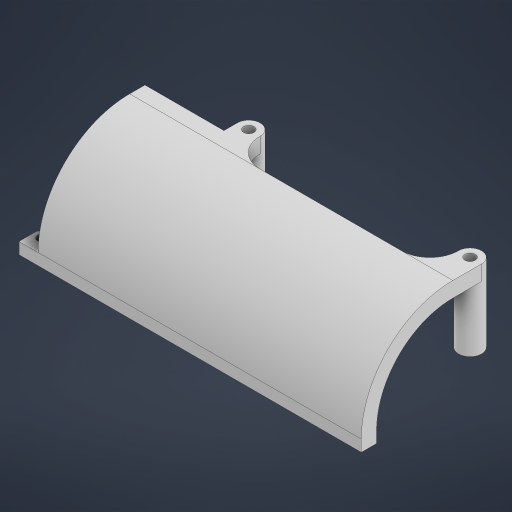
# Autodesk Inventor part: horizental blade
Saved by Autodesk Inventor 2024 (Build 280153000, 153)
## iProperties
Created: 2023-07-13
Part Number: horizental blade
Material: 일반
Document SubType Name: Modeling
Designer: 6gioc
Density: 1 g/cm^3
Appearance: 기본값
Author: 6gioc
Autodesk Inventor part; units mm, degrees
ref_plane "YZ Plane" through (0, 0, 0) normal (1, 0, 0) x (0, 1, 0)
ref_plane "XZ Plane" through (0, 0, 0) normal (0, 1, 0) x (-1, 0, 0)
ref_plane "XY Plane" through (0, 0, 0) normal (0, 0, 1) x (1, 0, 0)
sketch "스케치1" plane through (0, 0, 0) normal (0, 1, 0) x (-1, 0, 0)
  circle A0 centre (0, 0) radius 1.5
  circle A1 centre (0, 0) radius 2.5
  line L0 (2.5, 0) -> (2.5, 4)
  line L1 (2.5, 4) -> (-82.5, 4)
  line L2 (-82.5, 4) -> (-82.5, 0)
  line L3 (-82.5, 0) -> (-2.5, 0)
  line L4 (0, -2.5) -> (-5, -2.5)
  line L5 (-5, -2.5) -> (-7.5, 0)
  dimension "d0" = 3
  dimension "d1" = 5
  dimension "d2" = 4
  dimension "d3" = 85
  dimension "d4" = 5
  dimension "d5" = 135
  constraints: 12 end point, 3 perpendicular, 3 point on circle, 2 centre point, 2 coincident, 2 tangent, 1 horizontal, 1 point on line, 1 vertical
  measures "d0" diameter of A0
  measures "d1" diameter of A1
  measures "d2" distance of L0.start L0.end
  measures "d3" distance of L0.end L1.end
  measures "d4" distance of L4.start L4.end
  measures "d5" angle of L4 L5
extrude "돌출1" add sketch "스케치1" along normal blind 3
sketch "스케치2" plane through (82.5, 0, 4) normal (1, 0, 0) x (0, 0, -1)
  line L0 (4, 3) -> (24, 3)
  arc A0 (24, 27) -> (0, 3) centre (24, 3) ccw
  arc A1 (24, 23) -> (4, 3) centre (24, 3) ccw
  line L1 (24, 27) -> (24, 23)
  line L2 (0, 0) -> (4, 0) projected
  line L3 (4, 0) -> (4, 3) projected
  line L4 (0, 3) -> (4, 3) projected
  line L5 (0, 0) -> (0, 3) projected
  point P0 (4, 0)
  point P1 (0, 3)
  point P2 (4, 3)
  dimension "d8" = 20
  constraints: 4 end point, 4 point on circle, 2 centre point, 2 coincident, 1 horizontal
  measures "d8" distance of L0.start L0.end
extrude "돌출2" add sketch "스케치2" against normal blind 80 contours L1 A1 L4 A0
sketch "스케치3" plane through (82.5, 0, 4) normal (1, 0, 0) x (0, 0, -1)
  line L0 (0, 0) -> (4, 0) projected
  line L1 (4, 0) -> (4, 3) projected
  arc A0 (24, 23) -> (4, 3) centre (24, 3) ccw projected
  line L2 (24, 23) -> (24, 27) projected
  arc A1 (24, 27) -> (0, 3) centre (24, 3) ccw projected
  line L3 (0, 0) -> (0, 3) projected
  point P0 (4, 0)
extrude "돌출3" add sketch "스케치3" along normal blind 4.7
sketch "스케치4" plane through (2.5, 23, -20) normal (0, 0, -1) x (-1, 0, 0)
  line L0 (0, 4) -> (-84.7, 4) projected
  line L1 (-84.7, 4) -> (-78.7, 4)
  line L2 (-78.7, 4) -> (-78.7, 0)
  line L3 (-78.7, 0) -> (-84.7, 0)
  line L4 (-84.7, 0) -> (-84.7, 4)
  point P0 (2.5, -23)
  dimension "d16" = 6
  dimension "d17" = 4
  constraints: 8 end point, 2 parallel, 1 horizontal, 1 perpendicular
  measures "d16" distance of L2.end L3.end
  measures "d17" distance of L1.end L2.end
extrude "돌출4" add sketch "스케치4" along normal blind 10.5
sketch "스케치5" plane through (81.2, 23, -20) normal (0, -1, 0) x (1, 0, 0)
  circle A0 centre (3, -7.5) radius 1.35
  circle A1 centre (3, -7.5) radius 3
  line L0 (0, 0) -> (6, 0) projected
  line L1 (0, 0) -> (0, -10.5) projected
  line L2 (6, -10.5) -> (0, -10.5) projected
  line L3 (6, 0) -> (6, -10.5) projected
  line L4 (6, -10.5) -> (0, -10.5) projected
  line L5 (0, 0) -> (0, -10.5) projected
  point P0 (-81.2, 20)
  dimension "d20" = 2.7
  dimension "d21" = 6
  constraints: 2 centre point, 2 tangent, 1 coincident
  measures "d20" diameter of A0
  measures "d21" diameter of A1
extrude "돌출5" add sketch "스케치5" along normal blind 16.42 contours A1
fillet "모깎기1" radius 3 2 edges at (87.2, 25, -30.5) (81.2, 25, -30.5)
fillet "모깎기2" radius 7.5 1 edges at (81.2, 25, -20)
extrude "돌출6" cut sketch "스케치5" against normal blind 16.42 contours A0
sketch "스케치6" plane through (73.7, 23, -20) normal (0, 0, -1) x (-1, 0, 0)
  line L0 (71.2, 4) -> (0, 4) projected
  line L1 (50.5, 4) -> (44.5, 4)
  line L2 (44.5, 4) -> (44.5, 0)
  line L3 (44.5, 0) -> (50.5, 0)
  line L4 (50.5, 0) -> (50.5, 4)
  line L5 (-11.85, 4) -> (-9.15, 4) projected
  point P0 (73.7, -23)
  point P1 (51.2, 4)
  point P2 (47.5, 4)
  point P3 (-10.5, 4)
  point P4 (44.5, 4)
  dimension "d29" = 6
  dimension "d30" = 4
  dimension "d31" = 58
  constraints: 8 end point, 2 midpoint, 2 parallel, 1 horizontal, 1 perpendicular, 1 point on line
  measures "d29" distance of L3.end L2.end
  measures "d30" distance of L2.end L1.end
  measures "d31" distance of point (47.5, 4) point (-10.5, 4)
extrude "돌출7" add sketch "스케치6" along normal blind 10.5
sketch "스케치7" plane through (23.2, 27, -20) normal (0, 1, 0) x (1, 0, 0)
  circle A0 centre (3, 7.5) radius 1.35
  circle A1 centre (3, 7.5) radius 3
  line L0 (0, 0) -> (0, 10.5) projected
  line L1 (0, 10.5) -> (6, 10.5) projected
  point P0 (-23.2, -20)
  dimension "d34" = 2.7
  dimension "d35" = 6
  constraints: 2 centre point, 2 tangent, 1 coincident
  measures "d34" diameter of A0
  measures "d35" diameter of A1
extrude "돌출8" add sketch "스케치7" against normal blind 20.42 contours A1
extrude "돌출9" cut sketch "스케치7" against normal blind 20.42 contours A0
fillet "모깎기4" radius 3 2 edges at (23.2, 25, -30.5) (29.2, 25, -30.5)
fillet "모깎기6" radius 7.5 1 edges at (29.2, 25, -20)
sketch "스케치8" plane through (2.5, 23, -20) normal (0, 0, -1) x (-1, 0, 0)
  line L0 (-20.7, 4) -> (-20.7, 0) projected
  line L1 (0, 0) -> (-20.7, 0) projected
  line L2 (0, 4) -> (0, 0) projected
  line L3 (0, 4) -> (-20.7, 4) projected
  point P0 (2.5, -23)
extrude "돌출10" add sketch "스케치8" along normal blind 4
sketch "스케치9" plane through (2.5, 23, -20) normal (0, -1, 0) x (1, 0, 0)
  line L0 (0, -4) -> (20.7, -4) projected
  line L1 (0, -4) -> (20.7, -4)
  line L2 (20.7, -4) -> (20.7, -1)
  line L3 (20.7, -1) -> (0, -1)
  line L4 (0, -1) -> (0, -4)
  circle A0 centre (23.7, -7.5) radius 3 projected
  line L5 (25.6463, -5.2171) -> (20.7, -1)
  arc A1 (26.7, -7.5) -> (20.7, -7.5) centre (23.7, -7.5) ccw projected
  arc A2 (34.2, 0) -> (26.7, -7.5) centre (34.2, -7.5) ccw projected
  line L6 (0, 0) -> (34.2, 0) projected
  line L7 (0, 0) -> (0, -4) projected
  line L8 (20.7, -4) -> (0, -4) projected
  line L9 (20.7, -4) -> (20.7, -7.5) projected
  point P0 (-2.5, 20)
  dimension "d45" = 3
  constraints: 10 end point, 2 parallel, 1 horizontal, 1 perpendicular, 3 other
  measures "d45" distance of L2.end L0.end
extrude "돌출11" add sketch "스케치9" along normal blind 16.42 contours L4 L3 L2 L0
sketch "스케치10" plane through (2.5, 0, 4) normal (-1, 0, 0) x (0, 0, 1)
  arc A0 (0, 3) -> (-24, 27) centre (-24, 3) ccw projected
  line L0 (-24, 27) -> (-28, 27) projected
  line L1 (-24, 23) -> (-25, 23) projected
  arc A1 (-4, 3) -> (-24, 23) centre (-24, 3) ccw projected
  line L2 (-28, 27) -> (-28, 6.58) projected
  line L3 (-25, 6.58) -> (-28, 6.58) projected
  line L4 (-25, 23) -> (-25, 6.58) projected
  line L5 (-25, 6.58) -> (-4.2263, 6)
  line L6 (-25, 6.58) -> (-25, 0)
  line L7 (-25, 6.58) -> (-18.42, 6.58) construction
  line L8 (-4, 0) -> (-4, 3) projected
  line L9 (-25, 0) -> (-4, 0)
  arc A2 (-4, 3) -> (-24, 23) centre (-24, 3) ccw projected
  arc A3 (-4, 3) -> (-24, 23) centre (-24, 3) ccw projected
  line L10 (0, 3) -> (-4, 3) projected
  point P0 (-4, 3)
  point P1 (-4.2263, 6)
  dimension "d50" = 90
  constraints: 8 end point, 2 perpendicular, 1 horizontal
  measures "d50" angle of L6 L7
extrude "돌출12" add sketch "스케치10" against normal blind 3 contours L5 L4 L1 A1
sketch "스케치13" plane through (0, 3, 0) normal (0, 1, 0) x (1, 0, 0)
  line L0 (2.5, 0) -> (7.5, 0) projected
  line L1 (7.5, 0) -> (5, 2.5) projected
  line L2 (5, 2.5) -> (0, 2.5) projected
  arc A0 (0, 2.5) -> (-2.5, 0) centre (0, 0) ccw projected
  line L3 (-2.5, 0) -> (-2.5, -4) projected
  line L4 (-2.5, -4) -> (2.5, -4) projected
  line L5 (2.5, -4) -> (2.5, 0) projected
  circle A1 centre (0, 0) radius 1.5 projected
  line L6 (2.5, 20) -> (2.5, -4) projected
  line L7 (5.5, 0.2263) -> (5.5, 21) projected
  line L8 (5.5, 0.2263) -> (5.5, 0)
  line L9 (2.5, 0) -> (7.5, 0) projected
  line L10 (5.5, 0.2263) -> (5.7263, 0.2263) construction
  point P0 (5.5, 2)
  point P1 (2.5, 2.5)
  dimension "d53" = 90
  constraints: 4 end point, 1 horizontal, 1 perpendicular, 1 point on line
  measures "d53" angle of L8 L10
extrude "돌출14" add sketch "스케치13" along normal blind 3.5 contours L6 L2 L1 L7 L8 L0
chamfer "모따기2" distance 0.99 angle 45 4 edges at (6.5, 3, 0) (5.5, 3, -1) (5.5, 17.1421, -5.8579) (5.5, 23, -20.5)
chamfer "모따기3" distance 2 angle 45 1 edges at (5.5, 14.295, -21)
sketch "스케치14" plane through (2.5, 6.58, -20) normal (0, -1, 0) x (1, 0, 0)
  line L0 (0, 0) -> (0, -4) projected
  line L1 (5, -1) -> (20.7, -1) projected
  line L2 (0, -4) -> (5, -4)
  line L3 (5, -4) -> (5, -1)
  line L4 (5, -1) -> (0, -1)
  line L5 (0, -1) -> (0, -4)
  point P0 (-2.5, 20)
  point P1 (0, -1)
  dimension "d62" = 5
  dimension "d63" = 3
  constraints: 8 end point, 2 parallel, 1 horizontal, 1 perpendicular
  measures "d62" distance of L4.end L1.start
  measures "d63" distance of L1.start L2.end
extrude "돌출15" add sketch "스케치14" along normal blind 3
